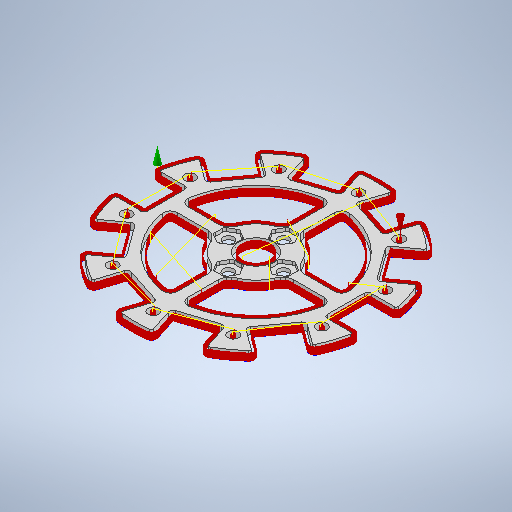
# Autodesk Inventor part: T2.0_base2
Saved by Autodesk Inventor 2025 (Build 290162000, 162)
## iProperties
Created: 2024-06-25
Part Number: T2.0_base2
Material: 一般
Document SubType Name: Modeling
Designer: 8326d
Density: 1 g/cm^3
Appearance: 既定
Author: 8326d
Autodesk Inventor part; units mm, degrees
ref_plane "YZ Plane" through (0, 0, 0) normal (1, 0, 0) x (0, 1, 0)
ref_plane "XZ Plane" through (0, 0, 0) normal (0, 1, 0) x (-1, 0, 0)
ref_plane "XY Plane" through (0, 0, 0) normal (0, 0, 1) x (1, 0, 0)
sketch "スケッチ1" plane through (0, 0, 0) normal (0, 1, 0) x (-1, 0, 0)
  circle A0 centre (0, 0) radius 35
  dimension "d0" = 70
  constraints: 1 centre point, 1 coincident
  measures "d0" diameter of A0
extrude "押し出し1" add sketch "スケッチ1" along normal blind 2
sketch "スケッチ2" plane through (0, 2, 0) normal (0, 1, 0) x (1, 0, 0)
  circle A0 centre (0, 0) radius 35 projected
  line L0 (-29.975, -8.2) -> (-33.025, -8.2)
  line L1 (-33.025, -8.2) -> (-33.025, 8.2)
  line L2 (-33.025, 8.2) -> (-29.975, 8.2)
  line L3 (-29.975, 8.2) -> (-29.975, -8.2)
  line L4 (-29.975, -8.2) -> (-33.025, 8.2) construction
  line L5 (-33.025, -8.2) -> (-29.975, 8.2) construction
  line L6 (-26, -6.3443) -> (-37, -6.3443)
  line L7 (-37, -6.3443) -> (-37, 6.3443)
  line L8 (-37, 6.3443) -> (-26, 6.3443)
  line L9 (-26, 6.3443) -> (-26, -6.3443)
  line L10 (-26, -6.3443) -> (-37, 6.3443) construction
  line L11 (-37, -6.3443) -> (-26, 6.3443) construction
  line L12 (-37, -6.3443) -> (0, 0) construction
  line L13 (0, 0) -> (-35, 0) construction
  point P0 (-31.5, 0)
  point P1 (-33.025, 6.3443)
  point P2 (-34.4202, 6.3443)
  point P3 (-34.4202, -6.3443)
  point P4 (-33.025, -6.3443)
  point P5 (-29.975, -6.3443)
  point P6 (-29.975, 6.3443)
  dimension "d3" = 31.5
  dimension "d4" = 16.4
  dimension "d5" = 3.05
  dimension "d6" = 9.73
  dimension "d7" = 2
  constraints: 28 end point, 4 midpoint, 4 parallel, 3 horizontal, 2 perpendicular, 1 horizontal alignment, 2 other
  measures "d3" distance of point (0, 0) point (-31.5, 0)
  measures "d4" distance of L0.end L1.end
  measures "d5" distance between parallel lines of L3 L1
  measures "d6" angle of L13 L12
  measures "d7" distance from line of L13.end L7
extrude "押し出し2" cut sketch "スケッチ2" against normal through all contours L8 L1 L6 A0 | L8 L3 L6 L1 | L8 L9 L6 L3
fillet "フィレット1" radius 1 2 edges at (-26, 1, 6.3443) (-26, 1, -6.3443)
pattern_circular "円形状パターン1" count 10 over 360 about axis through (0, -10, 0) along (0, 1, 0) of "押し出し2", "フィレット1"
sketch "スケッチ3" plane through (0, 2, 0) normal (0, 1, 0) x (1, 0, 0)
  point P0 (0, 0)
  point P1 (0, -29.75)
  dimension "d16" = 29.75
  constraints: 1 vertical alignment
  measures "d16" distance of point (0, 0) point (0, -29.75)
hole "穴1" at (0, 2, 29.75) direction (0, -1, 0) diameter 3.1 end through all
pattern_circular "円形状パターン2" count 10 over 360 about axis through (0, -10, 0) along (0, 1, 0) of "穴1"
fillet "フィレット5" radius 0.5 20 edges at (-16.6702, 1, 30.7751) (-24.1174, 1, 25.3643) (-4.6027, 1, 34.696) (4.6027, 1, 34.696) (16.6702, 1, 30.7751) (24.1174, 1, 25.3643) (31.5756, 1, 15.099) (34.4202, 1, 6.3443) (34.4202, 1, -6.3443) (31.5756, 1, -15.099) (24.1174, 1, -25.3643) (16.6702, 1, -30.7751) (4.6027, 1, -34.696) (-4.6027, 1, -34.696) (-16.6702, 1, -30.7751) (-24.1174, 1, -25.3643) (-31.5756, 1, -15.099) (-34.4202, 1, -6.3443) (-34.4202, 1, 6.3443) (-31.5756, 1, 15.099)
sketch "スケッチ4" plane through (0, 2, 0) normal (0, 1, 0) x (1, 0, 0)
  circle A0 centre (0, 0) radius 23.625
  circle A1 centre (0, 0) radius 10
  line L0 (-1.5, 9.8869) -> (-1.5, 23.5773)
  line L1 (0, 0) -> (-23.625, 0) construction
  line L2 (0, 0) -> (23.625, 0) construction
  line L3 (-9.8869, 1.5) -> (-23.5773, 1.5)
  circle A2 centre (0, 8) radius 3.5
  circle A3 centre (-8, 0) radius 3.5
  point P0 (-11.1623, 1.5)
  point P1 (-9.4844, 3.1696)
  point P2 (-3.1696, 9.4844)
  point P3 (-1.5, 11.1623)
  dimension "d29" = 47.25
  dimension "d30" = 20
  dimension "d31" = 180
  dimension "d32" = 1.5
  dimension "d33" = 1.5
  dimension "d43" = 7
  dimension "d44" = 7
  dimension "d45" = 8
  dimension "d46" = 8
  constraints: 8 end point, 5 point on circle, 4 centre point, 2 coincident, 1 collinear, 1 horizontal, 1 parallel, 1 point on line, 1 vertical, 1 vertical alignment
  measures "d29" diameter of A0
  measures "d30" diameter of A1
  measures "d31" angle of L1 L2
  measures "d32" distance from line of point (0, 0) L0
  measures "d33" distance between parallel lines of L1 L3
  measures "d43" diameter of A2
  measures "d44" diameter of A3
  measures "d45" distance of point (0, 0) A2.centre
  measures "d46" distance of point (0, 0) A3.centre
extrude "押し出し4" cut sketch "スケッチ4" against normal through all contours L0 A2 A1 A3 L3 A0 picked at (-11.403, 15.1383)
fillet "フィレット4" radius 2 6 edges at (-23.5773, 1, -1.5) (-1.5, 1, -23.5773) (-11.1623, 1, -1.5) (-9.4844, 1, -3.1696) (-3.1696, 1, -9.4844) (-1.5, 1, -11.1623)
pattern_circular "円形状パターン3" count 4 over 360 about axis through (0, -10, 0) along (0, 1, 0) of "押し出し4", "フィレット4"
sketch "スケッチ5" plane through (0, 2, 0) normal (0, 1, 0) x (1, 0, 0)
  circle A0 centre (0, 0) radius 5.05
  dimension "d40" = 10.1
  constraints: 1 centre point, 1 coincident
  measures "d40" diameter of A0
extrude "押し出し5" cut sketch "スケッチ5" against normal through all
sketch "スケッチ6" plane through (0, 2, 0) normal (0, 1, 0) x (1, 0, 0)
  arc A0 (-2.2273, 10.6999) -> (-2.887, 9.9787) centre (0, 8) ccw projected
  arc A1 (-9.9787, 2.887) -> (-10.6999, 2.2273) centre (-8, 0) ccw projected
  arc A2 (-2.887, -9.9787) -> (-2.2273, -10.6999) centre (0, -8) ccw projected
  arc A3 (9.9787, -2.887) -> (10.6999, -2.2273) centre (8, 0) ccw projected
  point P0 (0, 0)
hole "穴2" at (0, 2, -8) at (-8, 2, 0) at (0, 2, 8) at (8, 2, 0) direction (0, -1, 0) diameter 3.1 end through all
sketch "スケッチ8" plane through (0, 2, 0) normal (0, 1, 0) x (1, 0, 0)
  circle A0 centre (-8, 0) radius 1.55 projected
  line L0 (-8, -3.2332) -> (-10.8, -1.6166)
  line L1 (-10.8, -1.6166) -> (-10.8, 1.6166)
  line L2 (-10.8, 1.6166) -> (-8, 3.2332)
  line L3 (-8, 3.2332) -> (-5.2, 1.6166)
  line L4 (-5.2, 1.6166) -> (-5.2, -1.6166)
  line L5 (-5.2, -1.6166) -> (-8, -3.2332)
  line L6 (-8, -3.2332) -> (-8, 3.2332) construction
  line L7 (-5.2, 1.6166) -> (-10.8, -1.6166) construction
  line L8 (-5.2, -1.6166) -> (-10.8, 1.6166) construction
  circle A1 centre (-10.3237, -1.3416) radius 0.55
  circle A2 centre (-8, -2.6832) radius 0.55
  circle A3 centre (-5.6763, -1.3416) radius 0.55
  circle A4 centre (-5.6763, 1.3416) radius 0.55
  circle A5 centre (-8, 2.6832) radius 0.55
  circle A6 centre (-10.3237, 1.3416) radius 0.55
  point P0 (0, 0)
  point P1 (-10.3237, -1.8916)
  point P2 (-8.4763, -2.9582)
  point P3 (-7.5237, -2.9582)
  point P4 (-5.6763, -1.8916)
  point P5 (-5.2, -1.0666)
  point P6 (-5.2, 1.0666)
  point P7 (-5.6763, 1.8916)
  point P8 (-7.5237, 2.9582)
  point P9 (-8.4763, 2.9582)
  point P10 (-10.3237, 1.8916)
  point P11 (-10.8, 1.0666)
  point P12 (-10.8, -1.0666)
  dimension "d62" = 1.1
  dimension "d63" = 1.1
  dimension "d64" = 1.1
  dimension "d65" = 1.1
  dimension "d66" = 1.1
  dimension "d67" = 1.1
  dimension "d61" = 5.6
  constraints: 18 end point, 6 point on line, 1 coincident, 1 vertical, 1 vertical alignment, 31 other
  measures "d61" distance between parallel lines of L4 L1
extrude "押し出し7" cut sketch "スケッチ8" against normal blind 1 contours A0 | A2 L0 | L0 A2 L5 | L5 A2 | L0 A1 L1 A6 L2 A5 L3 A4 L4 A3 L5 A2 | A1 L0 | L0 L1 A1 | A3 L4 L5 | L5 A3 | A1 L1 | L4 A3 | A4 L3 L4 | L4 A4 | A6 L1 | L1 L2 A6 | L3 A4 | A6 L2 | A5 L2 L3 | L3 A5 | L2 A5
pattern_circular "円形状パターン4" count 4 over 360 about axis through (0, -10, 0) along (0, 1, 0) of "押し出し7"
equation "\"d0\" = 2 * r"
equation "\"d3\" = 0.9 * r"
equation "\"d16\" = 0.85 * r"
equation "\"d29\" = 1.35 * r"
equation "\"d33\" = d32"
equation "\"d46\" = d45"
equation "\"r\" = 35"
